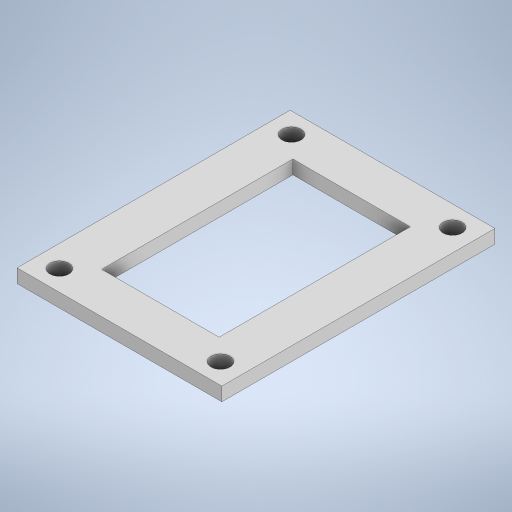
# Autodesk Inventor part: jetson_union
Saved by Autodesk Inventor 2023 (Build 270158000, 158)
## iProperties
Created: 2022-12-26
Part Number: jetson_union
Material: Genérico
Document SubType Name: Modeling
Designer: inigo
Density: 1 g/cm^3
Appearance: Valor por defecto
Author: inigo
Autodesk Inventor part; units mm, degrees
ref_plane "YZ Plane" through (0, 0, 0) normal (1, 0, 0) x (0, 1, 0)
ref_plane "XZ Plane" through (0, 0, 0) normal (0, 1, 0) x (-1, 0, 0)
ref_plane "XY Plane" through (0, 0, 0) normal (0, 0, 1) x (1, 0, 0)
sketch "Boceto1" plane through (0, 0, 0) normal (0, 1, 0) x (-1, 0, 0)
  circle A0 centre (-88.569, 59.1067) radius 3.5
  circle A1 centre (-29.569, 59.1067) radius 3.5
  line L0 (-88.569, 59.1067) -> (-29.569, 59.1067)
  circle A2 centre (-29.569, -25.8933) radius 3.5
  line L1 (-29.569, 59.1067) -> (-29.569, -25.8933)
  circle A3 centre (-88.569, -25.8933) radius 3.5
  line L2 (-29.569, -25.8933) -> (-88.569, -25.8933)
  line L3 (-88.569, -25.8933) -> (-88.569, 59.1067)
  line L4 (-96.569, 66.6067) -> (-21.569, 66.6067)
  line L5 (-21.569, 66.6067) -> (-21.569, 51.6067)
  line L6 (-96.569, 51.6067) -> (-96.569, 66.6067)
  line L7 (-96.569, 66.6067) -> (-21.569, 51.6067) construction
  line L8 (-21.569, 66.6067) -> (-96.569, 51.6067) construction
  line L9 (-37.569, -33.3933) -> (-21.569, -33.3933)
  line L10 (-21.569, -33.3933) -> (-21.569, 66.6067)
  line L11 (-21.569, 66.6067) -> (-37.569, 66.6067)
  line L12 (-37.569, -33.3933) -> (-21.569, 66.6067) construction
  line L13 (-21.569, -33.3933) -> (-37.569, 66.6067) construction
  line L14 (-21.569, -18.3933) -> (-21.569, -33.3933)
  line L15 (-21.569, -33.3933) -> (-96.569, -33.3933)
  line L16 (-96.569, -33.3933) -> (-96.569, -18.3933)
  line L17 (-96.569, -18.3933) -> (-21.569, -33.3933) construction
  line L18 (-21.569, -18.3933) -> (-96.569, -33.3933) construction
  line L19 (-80.569, -33.3933) -> (-96.569, -33.3933)
  line L20 (-96.569, -33.3933) -> (-96.569, 66.6067)
  line L21 (-96.569, 66.6067) -> (-80.569, 66.6067)
  line L22 (-80.569, -33.3933) -> (-96.569, 66.6067) construction
  line L23 (-96.569, -33.3933) -> (-80.569, 66.6067) construction
  line L24 (-80.569, -18.3933) -> (-37.569, -18.3933)
  line L25 (-80.569, 51.6067) -> (-80.569, -18.3933)
  line L26 (-37.569, 51.6067) -> (-37.569, -18.3933)
  circle A4 centre (-88.569, 59.1067) radius 3.5
  circle A5 centre (-29.569, 59.1067) radius 3.5
  circle A6 centre (-29.569, -25.8933) radius 3.5
  circle A7 centre (-88.569, -25.8933) radius 3.5
  line L27 (-37.569, 51.6067) -> (-80.569, 51.6067)
  point P0 (0, 0)
  point P1 (-59.069, 59.1067)
  point P2 (-29.569, 16.6067)
  point P3 (-59.069, -25.8933)
  point P4 (-88.569, 16.6067)
  dimension "d0" = 75
  dimension "d1" = 15
  constraints: 56 end point, 12 midpoint, 8 centre point, 8 parallel, 7 perpendicular, 4 coincident, 4 horizontal, 1 concentric
  measures "d0" distance of L7.end L6.start
  measures "d1" distance of L4.end L7.end
extrude "Extrusión1" add sketch "Boceto1" along normal blind 5 contours L0 A1 L1 A2 L2 A3 L3 A0 | L4 L5 L10 L9 L15 L16 L20 L6
